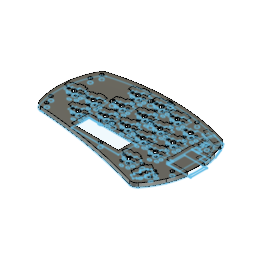
wubmeat-front (Autodesk Fusion 360 design; units mm, degrees)
Autodesk Fusion 360 part; units mm, degrees
(part 1 of 3)
sketch "Sketch1" plane through (0, 0, 0) normal (0, 0, 1) x (1, 0, 0)
  spline S0 degree 3 poles (91.4694, -71.3335) (91.4694, -70.9993) (91.6021, -70.6788) (91.8384, -70.4425) knots 0 0 0 0 1 1 1 1
  line L0 (93.9894, -71.3335) -> (93.9894, -71.3335)
  spline S1 degree 3 poles (103.5273, -74.6924) (103.1931, -74.6924) (102.8726, -74.5596) (102.6363, -74.3233) knots 0 0 0 0 1 1 1 1
  spline S2 degree 3 poles (16.5442, -44.4964) (16.5875, -44.9911) (17.0233, -45.3572) (17.5181, -45.3146) knots 0 0 0 0 1 1 1 1
  line L1 (38.2362, -60.5669) -> (36.9312, -60.6811)
  spline S3 degree 3 poles (61.5612, -48.3605) (61.9831, -48.7824) (62.2202, -49.3547) (62.2202, -49.9515) knots 0 0 0 0 1 1 1 1
  spline S4 degree 3 poles (59.9702, -47.7015) (60.5669, -47.7015) (61.1392, -47.9385) (61.5612, -48.3605) knots 0 0 0 0 1 1 1 1
  spline S5 degree 3 poles (39.0532, -59.592) (39.0099, -59.0973) (38.5741, -58.7311) (38.0794, -58.7738) knots 0 0 0 0 1 1 1 1
  line L2 (38.0794, -58.7738) -> (36.7744, -58.8879)
  spline S6 degree 3 poles (112.7726, -52.689) (113.0089, -52.9253) (113.1417, -53.2458) (113.1417, -53.58) knots 0 0 0 0 1 1 1 1
  spline S7 degree 3 poles (101.7793, -52.3051) (102.0156, -52.5414) (102.1483, -52.8619) (102.1483, -53.1961) knots 0 0 0 0 1 1 1 1
  spline S8 degree 3 poles (59.9702, -52.2015) (59.3735, -52.2015) (58.8012, -51.9644) (58.3792, -51.5425) knots 0 0 0 0 1 1 1 1
  spline S9 degree 3 poles (112.7726, -54.4709) (112.5363, -54.7072) (112.2158, -54.84) (111.8816, -54.84) knots 0 0 0 0 1 1 1 1
  line L3 (113.1417, -53.58) -> (113.1417, -53.58)
  spline S10 degree 3 poles (95.477, -77.878) (95.3823, -78.3656) (95.7004, -78.8377) (96.1878, -78.933) knots 0 0 0 0 1 1 1 1
  spline S11 degree 3 poles (110.6217, -53.58) (110.6217, -53.2458) (110.7544, -52.9253) (110.9907, -52.689) knots 0 0 0 0 1 1 1 1
  spline S12 degree 3 poles (93.6203, -72.2244) (93.384, -72.4607) (93.0635, -72.5935) (92.7294, -72.5935) knots 0 0 0 0 1 1 1 1
  spline S13 degree 3 poles (104.7873, -73.4324) (104.7873, -73.7666) (104.6545, -74.0871) (104.4182, -74.3233) knots 0 0 0 0 1 1 1 1
  spline S14 degree 3 poles (93.6203, -70.4425) (93.8566, -70.6788) (93.9894, -70.9993) (93.9894, -71.3335) knots 0 0 0 0 1 1 1 1
  spline S15 degree 3 poles (102.6363, -74.3233) (102.4, -74.0871) (102.2673, -73.7666) (102.2673, -73.4324) knots 0 0 0 0 1 1 1 1
  spline S16 degree 3 poles (17.3612, -43.5214) (16.8665, -43.5654) (16.5009, -44.0016) (16.5442, -44.4964) knots 0 0 0 0 1 1 1 1
  spline S17 degree 3 poles (111.8816, -54.84) (111.5475, -54.84) (111.227, -54.7072) (110.9907, -54.4709) knots 0 0 0 0 1 1 1 1
  line L4 (18.6662, -43.4073) -> (17.3612, -43.5214)
  spline S18 degree 3 poles (80.6112, -29.3105) (81.0331, -29.7324) (81.2702, -30.3047) (81.2702, -30.9015) knots 0 0 0 0 1 1 1 1
  spline S19 degree 3 poles (110.9907, -52.689) (111.227, -52.4527) (111.5475, -52.32) (111.8816, -52.32) knots 0 0 0 0 1 1 1 1
  spline S20 degree 3 poles (36.7744, -58.8879) (36.2797, -58.9319) (35.9141, -59.3681) (35.9574, -59.8629) knots 0 0 0 0 1 1 1 1
  spline S21 degree 3 poles (104.4182, -74.3233) (104.1819, -74.5596) (103.8614, -74.6924) (103.5273, -74.6924) knots 0 0 0 0 1 1 1 1
  line L5 (18.8231, -45.2004) -> (17.5181, -45.3146)
  spline S22 degree 3 poles (79.0202, -28.6515) (79.6169, -28.6515) (80.1892, -28.8885) (80.6112, -29.3105) knots 0 0 0 0 1 1 1 1
  spline S23 degree 3 poles (92.7294, -70.0735) (93.0635, -70.0735) (93.384, -70.2062) (93.6203, -70.4425) knots 0 0 0 0 1 1 1 1
  spline S24 degree 3 poles (19.6401, -44.2255) (19.5968, -43.7308) (19.161, -43.3646) (18.6662, -43.4073) knots 0 0 0 0 1 1 1 1
  spline S25 degree 3 poles (28.0789, -49.5101) (28.2116, -49.4999) (28.3345, -49.4367) (28.42, -49.3348) knots 0 0 0 0 1 1 1 1
  spline S26 degree 3 poles (38.2362, -60.5669) (38.7309, -60.523) (39.0965, -60.0867) (39.0532, -59.592) knots 0 0 0 0 1 1 1 1
  spline S27 degree 3 poles (81.2702, -30.9015) (81.2702, -31.4982) (81.0331, -32.0705) (80.6112, -32.4925) knots 0 0 0 0 1 1 1 1
  spline S28 degree 3 poles (110.9907, -54.4709) (110.7544, -54.2346) (110.6217, -53.9142) (110.6217, -53.58) knots 0 0 0 0 1 1 1 1
  spline S29 degree 3 poles (61.5612, -51.5425) (61.1392, -51.9644) (60.5669, -52.2015) (59.9702, -52.2015) knots 0 0 0 0 1 1 1 1
  line L6 (62.2202, -49.9515) -> (62.2202, -49.9515)
  spline S30 degree 3 poles (62.2202, -49.9515) (62.2202, -50.5482) (61.9831, -51.1205) (61.5612, -51.5425) knots 0 0 0 0 1 1 1 1
  spline S31 degree 3 poles (80.6112, -32.4925) (80.1892, -32.9144) (79.6169, -33.1515) (79.0202, -33.1515) knots 0 0 0 0 1 1 1 1
  spline S32 degree 3 poles (31.9578, -53.6879) (31.2089, -53.7176) (30.6072, -54.3153) (30.5725, -55.0639) knots 0 0 0 0 1 1 1 1
  spline S33 degree 3 poles (76.7702, -30.9015) (76.7702, -30.3047) (77.0073, -29.7324) (77.4292, -29.3105) knots 0 0 0 0 1 1 1 1
  spline S34 degree 3 poles (111.8816, -52.32) (112.2158, -52.32) (112.5363, -52.4527) (112.7726, -52.689) knots 0 0 0 0 1 1 1 1
  line L7 (102.1483, -53.1961) -> (102.1483, -53.1961)
  spline S35 degree 3 poles (35.9574, -59.8629) (36.0006, -60.3576) (36.4365, -60.7237) (36.9312, -60.6811) knots 0 0 0 0 1 1 1 1
  spline S36 degree 3 poles (102.2673, -73.4324) (102.2673, -73.0982) (102.4, -72.7777) (102.6363, -72.5414) knots 0 0 0 0 1 1 1 1
  spline S37 degree 3 poles (28.42, -49.3348) (28.5055, -49.2329) (28.5464, -49.1008) (28.5335, -48.9684) knots 0 0 0 0 1 1 1 1
  line L8 (33.5517, -53.5485) -> (31.9578, -53.6879)
  spline S38 degree 3 poles (58.3792, -51.5425) (57.9573, -51.1205) (57.7202, -50.5482) (57.7202, -49.9515) knots 0 0 0 0 1 1 1 1
  spline S39 degree 3 poles (58.3792, -48.3605) (58.8012, -47.9385) (59.3735, -47.7015) (59.9702, -47.7015) knots 0 0 0 0 1 1 1 1
  spline S40 degree 3 poles (96.5313, -77.1661) (96.0436, -77.0718) (95.5718, -77.3905) (95.477, -77.878) knots 0 0 0 0 1 1 1 1
  line L9 (97.4738, -79.183) -> (96.1878, -78.933)
  spline S41 degree 3 poles (77.4292, -32.4925) (77.0073, -32.0705) (76.7702, -31.4982) (76.7702, -30.9015) knots 0 0 0 0 1 1 1 1
  spline S42 degree 3 poles (91.8384, -72.2244) (91.6021, -71.9882) (91.4694, -71.6677) (91.4694, -71.3335) knots 0 0 0 0 1 1 1 1
  spline S43 degree 3 poles (91.8384, -70.4425) (92.0747, -70.2062) (92.3952, -70.0735) (92.7294, -70.0735) knots 0 0 0 0 1 1 1 1
  spline S44 degree 3 poles (99.6283, -53.1961) (99.6283, -52.5002) (100.1925, -51.9361) (100.8883, -51.9361) knots 0 0 0 0 1 1 1 1
  spline S45 degree 3 poles (57.7202, -49.9515) (57.7202, -49.3547) (57.9573, -48.7824) (58.3792, -48.3605) knots 0 0 0 0 1 1 1 1
  spline S46 degree 3 poles (79.0202, -33.1515) (78.4235, -33.1515) (77.8512, -32.9144) (77.4292, -32.4925) knots 0 0 0 0 1 1 1 1
  spline S47 degree 3 poles (92.7294, -72.5935) (92.3952, -72.5935) (92.0747, -72.4607) (91.8384, -72.2244) knots 0 0 0 0 1 1 1 1
  spline S48 degree 3 poles (93.9894, -71.3335) (93.9894, -71.6677) (93.8566, -71.9882) (93.6203, -72.2244) knots 0 0 0 0 1 1 1 1
  line L10 (21.1311, -51.2724) -> (23.6963, -51.0479)
  spline S49 degree 3 poles (113.1417, -53.58) (113.1417, -53.9142) (113.0089, -54.2346) (112.7726, -54.4709) knots 0 0 0 0 1 1 1 1
  spline S50 degree 3 poles (77.4292, -29.3105) (77.8512, -28.8885) (78.4235, -28.6515) (79.0202, -28.6515) knots 0 0 0 0 1 1 1 1
  line L11 (81.2702, -30.9015) -> (81.2702, -30.9015)
  line L12 (97.8172, -77.4161) -> (96.5313, -77.1661)
  line L13 (30.6553, -56.0103) -> (30.5725, -55.0639)
  line L14 (78.4006, -7.8462) -> (80.9752, -7.8911)
  line L15 (32.9635, -30.5322) -> (33.0053, -31.0104)
  spline S51 degree 3 poles (88.9155, -11.3802) (88.1676, -11.3315) (87.5067, -11.8629) (87.3939, -12.6039) knots 0 0 0 0 1 1 1 1
  spline S52 degree 3 poles (93.1621, -17.0552) (92.6655, -17.047) (92.2561, -17.4428) (92.2474, -17.9394) knots 0 0 0 0 1 1 1 1
  line L16 (23.6963, -51.0479) -> (23.5961, -49.9023)
  line L17 (94.5104, -10.5778) -> (94.5906, -5.9785)
  line L18 (80.9953, -6.7413) -> (85.4946, -6.8198)
  line L19 (35.9565, -35.3697) -> (35.5556, -30.7872)
  line L20 (22.6156, -38.6951) -> (20.0504, -38.9196)
  line L21 (22.2146, -34.1126) -> (22.1144, -32.967)
  line L22 (19.6494, -34.3371) -> (22.2146, -34.1126)
  spline S53 degree 3 poles (92.2474, -17.9394) (92.2387, -18.436) (92.6341, -18.8458) (93.1307, -18.8549) knots 0 0 0 0 1 1 1 1
  line L23 (22.6984, -39.6415) -> (22.6156, -38.6951)
  line L24 (94.4405, -18.8778) -> (93.1307, -18.8549)
  line L25 (80.8783, -13.4403) -> (80.8949, -12.4904)
  line L26 (33.0053, -31.0104) -> (35.5556, -30.7872)
  line L27 (86.0207, -5.3288) -> (86.5293, -4.8376)
  spline S54 degree 3 poles (94.4405, -18.8778) (94.9371, -18.886) (95.3465, -18.4903) (95.3552, -17.9936) knots 0 0 0 0 1 1 1 1
  line L28 (29.1736, -39.075) -> (22.6984, -39.6415)
  line L29 (91.5286, -4.9249) -> (92.0394, -5.4539)
  line L30 (92.0394, -5.4539) -> (92.031, -5.9338)
  line L31 (86.0032, -6.3286) -> (86.0207, -5.3288)
  line L32 (80.9752, -7.8911) -> (80.9953, -6.7413)
  line L33 (20.0504, -38.9196) -> (19.6494, -34.3371)
  line L34 (24.18, -56.5768) -> (24.0972, -55.6304)
  line L35 (28.4463, -47.9722) -> (28.9008, -47.4306)
  line L36 (91.4808, -10.5249) -> (90.5153, -11.4082)
  line L37 (27.4192, -30.4953) -> (32.4001, -30.0595)
  line L38 (27.0518, -32.0331) -> (26.9646, -31.0369)
  line L39 (34.4451, -47.4675) -> (34.487, -47.9457)
  line L40 (24.0972, -55.6304) -> (21.532, -55.8549)
  spline S55 degree 3 poles (95.3552, -17.9936) (95.3639, -17.497) (94.9685, -17.0872) (94.4719, -17.0781) knots 0 0 0 0 1 1 1 1
  line L41 (33.8818, -46.9948) -> (34.4451, -47.4675)
  line L42 (30.6553, -56.0103) -> (24.18, -56.5768)
  line L43 (21.532, -55.8549) -> (21.1311, -51.2724)
  line L44 (34.4197, -52.5691) -> (33.5517, -53.5485)
  line L45 (78.3203, -12.4455) -> (78.4006, -7.8462)
  line L46 (32.938, -35.6338) -> (32.0701, -36.6132)
  line L47 (29.1736, -39.075) -> (29.0908, -38.1286)
  line L48 (28.9008, -47.4306) -> (33.8818, -46.9948)
  line L49 (28.5335, -48.9684) -> (28.4463, -47.9722)
  line L50 (22.1144, -32.967) -> (26.5973, -32.5748)
  line L51 (35.9565, -35.3697) -> (32.938, -35.6338)
  spline S56 degree 3 poles (35.2927, -41.9526) (34.798, -41.9965) (34.4324, -42.4328) (34.4757, -42.9275) knots 0 0 0 0 1 1 1 1
  line L52 (32.4001, -30.0595) -> (32.9635, -30.5322)
  spline S57 degree 3 poles (30.4762, -36.7526) (29.7273, -36.7823) (29.1256, -37.3799) (29.0908, -38.1286) knots 0 0 0 0 1 1 1 1
  spline S58 degree 3 poles (26.5973, -32.5748) (26.7299, -32.5646) (26.8529, -32.5014) (26.9384, -32.3995) knots 0 0 0 0 1 1 1 1
  line L53 (32.0701, -36.6132) -> (30.4762, -36.7526)
  line L54 (37.4381, -52.305) -> (34.4197, -52.5691)
  spline S59 degree 3 poles (85.4946, -6.8198) (85.6276, -6.8235) (85.7564, -6.7735) (85.8521, -6.6811) knots 0 0 0 0 1 1 1 1
  line L55 (86.5293, -4.8376) -> (91.5286, -4.9249)
  line L56 (23.5961, -49.9023) -> (28.0789, -49.5101)
  line L57 (87.3773, -13.5537) -> (80.8783, -13.4403)
  line L58 (92.031, -5.9338) -> (94.5906, -5.9785)
  spline S60 degree 3 poles (26.9384, -32.3995) (27.0239, -32.2976) (27.0648, -32.1655) (27.0518, -32.0331) knots 0 0 0 0 1 1 1 1
  line L59 (34.487, -47.9457) -> (37.0372, -47.7225)
  line L60 (80.8949, -12.4904) -> (78.3203, -12.4455)
  spline S61 degree 3 poles (85.8521, -6.6811) (85.9478, -6.5887) (86.0023, -6.4617) (86.0032, -6.3286) knots 0 0 0 0 1 1 1 1
  line L61 (94.4719, -17.0781) -> (93.1621, -17.0552)
  line L62 (87.3773, -13.5537) -> (87.3939, -12.6039)
  line L63 (90.5153, -11.4082) -> (88.9155, -11.3802)
  line L64 (94.5104, -10.5778) -> (91.4808, -10.5249)
  line L65 (37.4381, -52.305) -> (37.0372, -47.7225)
  spline S62 degree 3 poles (104.0916, -28.9482) (104.1889, -28.8574) (104.2456, -28.7314) (104.2488, -28.5984) knots 0 0 0 0 1 1 1 1
  line L66 (112.6805, -32.9953) -> (112.8411, -28.3981)
  line L67 (104.8009, -27.1167) -> (109.7978, -27.2912)
  spline S63 degree 3 poles (107.0725, -33.7) (106.3256, -33.6382) (105.6555, -34.1581) (105.5298, -34.8969) knots 0 0 0 0 1 1 1 1
  spline S64 degree 3 poles (37.5716, -42.6567) (37.5283, -42.162) (37.0925, -41.7958) (36.5977, -41.8385) knots 0 0 0 0 1 1 1 1
  line L68 (112.6805, -32.9953) -> (109.6524, -32.8896)
  line L69 (99.0338, -34.6701) -> (96.4603, -34.5802)
  line L70 (96.4603, -34.5802) -> (96.6209, -29.983)
  line L71 (36.5977, -41.8385) -> (35.2927, -41.9526)
  spline S65 degree 3 poles (103.7317, -29.0806) (103.8646, -29.0866) (103.9943, -29.0389) (104.0916, -28.9482) knots 0 0 0 0 1 1 1 1
  line L72 (105.4967, -35.8463) -> (105.5298, -34.8969)
  spline S66 degree 3 poles (34.4757, -42.9275) (34.519, -43.4223) (34.9548, -43.7884) (35.4496, -43.7458) knots 0 0 0 0 1 1 1 1
  line L73 (108.6715, -33.7559) -> (107.0725, -33.7)
  line L74 (110.2994, -27.8291) -> (110.2826, -28.3088)
  line L75 (99.2344, -28.9236) -> (103.7317, -29.0806)
  line L76 (112.5286, -39.494) -> (111.2194, -39.4483)
  spline S67 degree 3 poles (112.4658, -41.2929) (112.9623, -41.3099) (113.3787, -40.9213) (113.396, -40.4248) knots 0 0 0 0 1 1 1 1
  line L77 (112.4658, -41.2929) -> (111.1566, -41.2472)
  spline S68 degree 3 poles (110.2894, -40.3163) (110.2721, -40.8128) (110.6602, -41.2294) (111.1566, -41.2472) knots 0 0 0 0 1 1 1 1
  spline S69 degree 3 poles (113.0591, -24.3032) (113.5556, -24.3202) (113.972, -23.9317) (113.9893, -23.4352) knots 0 0 0 0 1 1 1 1
  spline S70 degree 3 poles (113.9893, -23.4352) (114.0067, -22.9387) (113.6184, -22.522) (113.1219, -22.5043) knots 0 0 0 0 1 1 1 1
  line L78 (110.8759, -11.3191) -> (113.4344, -11.4085)
  line L79 (104.877, -10.6093) -> (105.3942, -10.1271)
  line L80 (109.7978, -27.2912) -> (110.2994, -27.8291)
  spline S71 degree 3 poles (36.7546, -43.6316) (37.2493, -43.5877) (37.6149, -43.1514) (37.5716, -42.6567) knots 0 0 0 0 1 1 1 1
  line L81 (109.6524, -32.8896) -> (108.6715, -33.7559)
  spline S72 degree 3 poles (111.2194, -39.4483) (110.723, -39.4314) (110.3068, -39.8199) (110.2894, -40.3163) knots 0 0 0 0 1 1 1 1
  spline S73 degree 3 poles (113.396, -40.4248) (113.4134, -39.9283) (113.0251, -39.5117) (112.5286, -39.494) knots 0 0 0 0 1 1 1 1
  line L82 (36.7546, -43.6316) -> (35.4496, -43.7458)
  line L83 (113.0591, -24.3032) -> (111.7499, -24.2575)
  line L84 (110.3911, -10.3016) -> (110.8927, -10.8394)
  line L85 (99.8277, -11.9339) -> (104.325, -12.091)
  line L86 (106.0899, -18.8567) -> (99.5939, -18.6299)
  spline S74 degree 3 poles (104.325, -12.091) (104.4579, -12.097) (104.5876, -12.0493) (104.6849, -11.9585) knots 0 0 0 0 1 1 1 1
  spline S75 degree 3 poles (110.8825, -23.3267) (110.8652, -23.8232) (111.2534, -24.2398) (111.7499, -24.2575) knots 0 0 0 0 1 1 1 1
  line L87 (113.2738, -16.0057) -> (113.4344, -11.4085)
  line L88 (106.0899, -18.8567) -> (106.1231, -17.9073)
  line L89 (99.0006, -35.6195) -> (99.0338, -34.6701)
  line L90 (99.5939, -18.6299) -> (99.6271, -17.6804)
  line L91 (97.2142, -12.9934) -> (99.7876, -13.0832)
  line L92 (110.2457, -15.8999) -> (109.2648, -16.7662)
  line L93 (26.9646, -31.0369) -> (27.4192, -30.4953)
  line L94 (105.4967, -35.8463) -> (99.0006, -35.6195)
  line L95 (110.2826, -28.3088) -> (112.8411, -28.3981)
  spline S76 degree 3 poles (107.6658, -16.7104) (106.9189, -16.6486) (106.2488, -17.1684) (106.1231, -17.9073) knots 0 0 0 0 1 1 1 1
  line L96 (99.7876, -13.0832) -> (99.8277, -11.9339)
  line L97 (113.1219, -22.5043) -> (111.8127, -22.4586)
  line L98 (104.2488, -28.5984) -> (104.2837, -27.599)
  line L99 (96.6209, -29.983) -> (99.1943, -30.0729)
  spline S77 degree 3 poles (104.6849, -11.9585) (104.7822, -11.8678) (104.8389, -11.7417) (104.8421, -11.6087) knots 0 0 0 0 1 1 1 1
  line L100 (109.2648, -16.7662) -> (107.6658, -16.7104)
  line L101 (104.2837, -27.599) -> (104.8009, -27.1167)
  line L102 (113.2738, -16.0057) -> (110.2457, -15.8999)
  line L103 (110.8927, -10.8394) -> (110.8759, -11.3191)
  line L104 (97.0536, -17.5906) -> (97.2142, -12.9934)
  spline S78 degree 3 poles (111.8127, -22.4586) (111.3162, -22.4416) (110.8998, -22.8302) (110.8825, -23.3267) knots 0 0 0 0 1 1 1 1
  line L105 (99.6271, -17.6804) -> (97.0536, -17.5906)
  line L106 (99.1943, -30.0729) -> (99.2344, -28.9236)
  spline S79 degree 3 poles (112.1172, -74.4556) (112.0677, -74.3829) (111.9997, -74.3248) (111.9203, -74.2871) knots 0 0 0 0 1 1 1 1
  line L107 (122.6316, -28.9815) -> (118.7816, -28.9815)
  line L108 (118.7816, -28.9815) -> (118.7816, -25.5915)
  spline S80 degree 3 poles (93.8471, -52.8726) (94.3438, -52.8808) (94.7531, -52.4851) (94.7618, -51.9885) knots 0 0 0 0 1 1 1 1
  line L109 (93.8785, -51.0729) -> (92.5687, -51.05)
  line L110 (93.917, -44.5726) -> (90.8874, -44.5197)
  spline S81 degree 3 poles (84.9012, -40.8147) (85.0342, -40.8184) (85.163, -40.7684) (85.2587, -40.6759) knots 0 0 0 0 1 1 1 1
  line L111 (116.1996, -81.9373) -> (115.3459, -81.5208)
  spline S82 degree 3 poles (112.2014, -74.701) (112.1957, -74.6132) (112.1666, -74.5284) (112.1172, -74.4556) knots 0 0 0 0 1 1 1 1
  line L112 (119.0491, -76.0948) -> (116.1996, -81.9373)
  line L113 (111.2113, -79.5044) -> (110.1778, -79)
  line L114 (118.0383, -71.0961) -> (118.4305, -72.3441)
  spline S83 degree 3 poles (117.5933, -74.8209) (117.6795, -75.1722) (117.8944, -75.4783) (118.1954, -75.6788) knots 0 0 0 0 1 1 1 1
  line L115 (112.9833, -68.6859) -> (113.6783, -68.4466)
  line L116 (105.3942, -10.1271) -> (110.3911, -10.3016)
  line L117 (118.4305, -72.3441) -> (117.7292, -73.7822)
  spline S84 degree 3 poles (91.654, -51.9342) (91.6454, -52.4309) (92.0407, -52.8406) (92.5373, -52.8498) knots 0 0 0 0 1 1 1 1
  line L118 (89.9219, -45.403) -> (88.3221, -45.3751)
  spline S85 degree 3 poles (127.7514, -8.5717) (124.8031, -7.6317) (121.8191, -6.8079) (118.8062, -6.1021) knots 0 0 0 0 1 1 1 1
  spline S86 degree 3 poles (127.9715, -8.6379) (127.8982, -8.6158) (127.8248, -8.5937) (127.7514, -8.5717) knots 0 0 0 0 1 1 1 1
  spline S87 degree 3 poles (112.1503, -74.9553) (112.1896, -74.8766) (112.2073, -74.7888) (112.2014, -74.701) knots 0 0 0 0 1 1 1 1
  line L119 (114.2168, -83.8348) -> (110.0827, -81.8184)
  line L120 (85.9359, -38.8324) -> (90.9352, -38.9197)
  spline S88 degree 3 poles (92.5687, -51.05) (92.0721, -51.0419) (91.6627, -51.4376) (91.654, -51.9342) knots 0 0 0 0 1 1 1 1
  line L121 (119.3664, -68.3727) -> (118.0383, -71.0961)
  line L122 (115.2322, -66.3558) -> (115.2322, -66.3558)
  line L123 (122.6316, -28.9815) -> (118.7816, -28.9815)
  line L124 (118.7816, -25.5915) -> (122.6316, -25.5915)
  line L125 (111.0216, -73.8484) -> (110.7912, -73.1802)
  line L126 (90.8874, -44.5197) -> (89.9219, -45.403)
  line L127 (110.7912, -73.1802) -> (112.9833, -68.6859)
  spline S89 degree 3 poles (85.2587, -40.6759) (85.3544, -40.5835) (85.4089, -40.4565) (85.4098, -40.3235) knots 0 0 0 0 1 1 1 1
  line L128 (118.8062, -6.1021) -> (118.8062, -6.1021)
  line L129 (85.4098, -40.3235) -> (85.4273, -39.3236)
  spline S90 degree 3 poles (117.7292, -73.7822) (117.5555, -74.0992) (117.507, -74.4699) (117.5933, -74.8209) knots 0 0 0 0 1 1 1 1
  line L130 (119.8516, -54.0815) -> (119.8516, -37.7315)
  line L131 (118.4516, -54.0665) -> (118.4516, -29.0465)
  line L132 (120.2166, -19.5965) -> (120.2166, -16.4365)
  line L133 (122.6316, -25.5915) -> (122.6316, -28.9815)
  line L134 (115.2322, -66.3558) -> (119.3664, -68.3727)
  line L135 (133.7216, -15.5315) -> (128.9416, -17.3815)
  line L136 (110.1778, -79) -> (112.1503, -74.9553)
  line L137 (114.1098, -68.657) -> (115.2322, -66.3558)
  line L138 (136.3216, -29.0465) -> (136.3216, -33.6665)
  spline S91 degree 3 poles (88.3221, -45.3751) (87.5742, -45.3263) (86.9134, -45.8578) (86.8005, -46.5987) knots 0 0 0 0 1 1 1 1
  line L139 (113.6783, -68.4466) -> (114.1098, -68.657)
  spline S92 degree 3 poles (94.7618, -51.9885) (94.7705, -51.4918) (94.3752, -51.0821) (93.8785, -51.0729) knots 0 0 0 0 1 1 1 1
  line L140 (118.1954, -75.6788) -> (119.0491, -76.0948)
  line L141 (91.4377, -39.9286) -> (93.9973, -39.9733)
  line L142 (104.8421, -11.6087) -> (104.877, -10.6093)
  line L143 (90.9352, -38.9197) -> (91.446, -39.4487)
  line L144 (86.784, -47.5486) -> (80.2849, -47.4351)
  line L145 (86.784, -47.5486) -> (86.8005, -46.5987)
  line L146 (110.0827, -81.8184) -> (111.2113, -79.5044)
  line L147 (93.8471, -52.8726) -> (92.5373, -52.8498)
  line L148 (115.3459, -81.5208) -> (114.2168, -83.8348)
  line L149 (111.9203, -74.2871) -> (111.0216, -73.8484)
  line L150 (118.7816, -28.9815) -> (118.7816, -25.5915)
  line L151 (118.7816, -25.5915) -> (122.6316, -25.5915)
  line L152 (137.2216, -24.2815) -> (133.7216, -15.5315)
  line L153 (119.0516, -48.9015) -> (119.0516, -52.5115)
  line L154 (115.5823, -12.1346) -> (111.6395, -11.0314)
  line L155 (119.8516, -54.0815) -> (119.8516, -37.7315)
  line L156 (123.5816, -25.9315) -> (123.5816, -29.0215)
  line L157 (123.5816, -29.0215) -> (125.0516, -29.0215)
  line L158 (118.6066, -16.4365) -> (118.6066, -19.5965)
  line L159 (116.5981, -7.8464) -> (115.5823, -12.1346)
  line L160 (112.695, -6.8695) -> (116.5981, -7.8464)
  line L161 (131.0416, -33.6665) -> (131.0416, -29.0465)
  line L162 (120.2166, -16.4365) -> (118.6066, -16.4365)
  line L163 (121.8916, -24.6315) -> (121.8916, -21.4715)
  line L164 (121.8916, -24.6315) -> (121.8916, -21.4715)
  line L165 (122.9416, -19.6115) -> (122.9416, -16.4515)
  spline S93 degree 3 poles (50.2132, -44.4132) (49.4637, -44.4168) (48.8415, -44.993) (48.7806, -45.74) knots 0 0 0 0 1 1 1 1
  line L166 (115.0116, -13.2315) -> (117.0316, -5.3565)
  line L167 (121.8916, -21.4715) -> (119.4916, -21.4715)
  line L168 (122.9416, -16.4515) -> (121.3316, -16.4515)
  line L169 (119.4916, -24.6315) -> (121.8916, -24.6315)
  line L170 (119.8516, -37.7315) -> (142.1616, -37.7315)
  line L171 (136.3216, -29.0465) -> (136.3216, -33.6665)
  line L172 (119.0516, -52.5115) -> (116.9616, -52.5115)
  line L173 (136.3216, -33.6665) -> (131.0416, -33.6665)
  line L174 (116.9616, -52.5115) -> (116.9616, -48.9015)
  line L175 (118.6066, -19.5965) -> (120.2166, -19.5965)
  line L176 (116.9616, -48.9015) -> (119.0516, -48.9015)
  line L177 (128.9416, -17.3815) -> (132.3216, -26.0915)
  line L178 (111.6395, -11.0314) -> (112.695, -6.8695)
  line L179 (118.4516, -29.0465) -> (131.1316, -29.0465)
  line L180 (116.9616, -48.9015) -> (119.0516, -48.9015)
  line L181 (119.0516, -52.5115) -> (116.9616, -52.5115)
  line L182 (129.5116, -8.7615) -> (127.3916, -16.5315)
  line L183 (121.3316, -19.6115) -> (122.9416, -19.6115)
  line L184 (127.3916, -16.5315) -> (115.0116, -13.2315)
  line L185 (142.1616, -37.7315) -> (142.1616, -54.0815)
  line L186 (136.3216, -33.6665) -> (131.0416, -33.6665)
  line L187 (131.1316, -54.0665) -> (118.4516, -54.0665)
  line L188 (119.8516, -37.7315) -> (142.1616, -37.7315)
  line L189 (118.6066, -19.5965) -> (120.2166, -19.5965)
  line L190 (131.0416, -29.0465) -> (136.3216, -29.0465)
  line L191 (120.2166, -19.5965) -> (120.2166, -16.4365)
  line L192 (142.1616, -54.0815) -> (119.8516, -54.0815)
  line L193 (131.1316, -54.0665) -> (118.4516, -54.0665)
  line L194 (118.4516, -54.0665) -> (118.4516, -29.0465)
  line L195 (118.4516, -29.0465) -> (131.1316, -29.0465)
  line L196 (119.0516, -48.9015) -> (119.0516, -52.5115)
  line L197 (120.2166, -16.4365) -> (118.6066, -16.4365)
  line L198 (131.0416, -29.0465) -> (136.3216, -29.0465)
  line L199 (117.0316, -5.3565) -> (129.5116, -8.7615)
  line L200 (142.1616, -54.0815) -> (119.8516, -54.0815)
  line L201 (131.1316, -29.0465) -> (131.1316, -54.0665)
  line L202 (125.0516, -29.0215) -> (125.0516, -25.9315)
  line L203 (119.4916, -21.4715) -> (119.4916, -24.6315)
  line L204 (121.3316, -16.4515) -> (121.3316, -19.6115)
  line L205 (125.0516, -25.9315) -> (123.5816, -25.9315)
  line L206 (125.0516, -29.0215) -> (125.0516, -25.9315)
  line L207 (122.9416, -19.6115) -> (122.9416, -16.4515)
  line L208 (48.8304, -46.6887) -> (48.7806, -45.74)
  line L209 (52.9161, -38.2834) -> (52.9412, -38.7627)
  line L210 (132.3216, -26.0915) -> (137.2216, -24.2815)
  line L211 (122.9416, -16.4515) -> (121.3316, -16.4515)
  spline S94 degree 3 poles (46.8294, -39.9393) (46.9185, -39.8404) (46.9639, -39.7099) (46.9556, -39.5771) knots 0 0 0 0 1 1 1 1
  line L212 (42.0488, -41.4865) -> (41.9886, -40.3381)
  line L213 (46.9033, -38.5785) -> (47.3764, -38.053)
  line L214 (39.7181, -46.215) -> (39.4773, -41.6213)
  line L215 (123.5816, -29.0215) -> (125.0516, -29.0215)
  line L216 (121.8916, -21.4715) -> (119.4916, -21.4715)
  line L217 (46.9556, -39.5771) -> (46.9033, -38.5785)
  line L218 (55.7384, -43.2224) -> (55.4977, -38.6287)
  line L219 (55.7384, -43.2224) -> (52.7126, -43.381)
  line L220 (42.2895, -46.0802) -> (39.7181, -46.215)
  line L221 (39.4773, -41.6213) -> (42.0488, -41.4865)
  line L222 (52.7126, -43.381) -> (51.811, -44.3295)
  line L223 (52.3696, -37.7913) -> (52.9161, -38.2834)
  line L224 (48.8304, -46.6887) -> (42.3393, -47.0289)
  line L225 (51.811, -44.3295) -> (50.2132, -44.4132)
  spline S95 degree 3 poles (57.0984, -50.5613) (57.0724, -50.0653) (56.6495, -49.6842) (56.1535, -49.7096) knots 0 0 0 0 1 1 1 1
  spline S96 degree 3 poles (56.2477, -51.5071) (56.7437, -51.4806) (57.1243, -51.0573) (57.0984, -50.5613) knots 0 0 0 0 1 1 1 1
  line L226 (52.9412, -38.7627) -> (55.4977, -38.6287)
  line L227 (41.9886, -40.3381) -> (46.4825, -40.1026)
  line L228 (56.1535, -49.7096) -> (54.8453, -49.7782)
  line L229 (125.0516, -25.9315) -> (123.5816, -25.9315)
  line L230 (121.3316, -19.6115) -> (122.9416, -19.6115)
  line L231 (42.3393, -47.0289) -> (42.2895, -46.0802)
  line L232 (47.3764, -38.053) -> (52.3696, -37.7913)
  spline S97 degree 3 poles (75.73, -32.7747) (76.0515, -32.7747) (76.3487, -32.6031) (76.5094, -32.3247) knots 0 0 0 0 1 1 1 1
  spline S98 degree 3 poles (46.4825, -40.1026) (46.6154, -40.097) (46.7404, -40.0381) (46.8294, -39.9393) knots 0 0 0 0 1 1 1 1
  line L233 (119.4916, -24.6315) -> (121.8916, -24.6315)
  line L234 (75.73, -32.7747) -> (74.42, -32.7747)
  spline S99 degree 3 poles (53.9947, -50.724) (54.0207, -51.2199) (54.4435, -51.6011) (54.9395, -51.5757) knots 0 0 0 0 1 1 1 1
  spline S100 degree 3 poles (76.5094, -31.4247) (76.3487, -31.1462) (76.0515, -30.9747) (75.73, -30.9747) knots 0 0 0 0 1 1 1 1
  spline S101 degree 3 poles (74.42, -30.9747) (74.0985, -30.9747) (73.8013, -31.1462) (73.6406, -31.4247) knots 0 0 0 0 1 1 1 1
  line L235 (126.8594, -71.9436) -> (126.2851, -73.1211)
  spline S102 degree 3 poles (73.6406, -32.3247) (73.8013, -32.6031) (74.0985, -32.7747) (74.42, -32.7747) knots 0 0 0 0 1 1 1 1
  spline S103 degree 3 poles (76.5094, -32.3247) (76.6702, -32.0462) (76.6702, -31.7031) (76.5094, -31.4247) knots 0 0 0 0 1 1 1 1
  line L236 (75.73, -30.9747) -> (74.42, -30.9747)
  spline S104 degree 3 poles (124.6673, -72.332) (124.4501, -72.7786) (124.6358, -73.3167) (125.0821, -73.5344) knots 0 0 0 0 1 1 1 1
  line L237 (56.2477, -51.5071) -> (54.9395, -51.5757)
  spline S105 degree 3 poles (126.445, -70.7402) (125.9982, -70.5224) (125.4594, -70.7079) (125.2415, -71.1546) knots 0 0 0 0 1 1 1 1
  spline S106 degree 3 poles (54.8453, -49.7782) (54.3494, -49.8047) (53.9687, -50.228) (53.9947, -50.724) knots 0 0 0 0 1 1 1 1
  spline S107 degree 3 poles (73.6406, -31.4247) (73.4798, -31.7031) (73.4798, -32.0462) (73.6406, -32.3247) knots 0 0 0 0 1 1 1 1
  spline S108 degree 3 poles (126.8594, -71.9436) (127.0772, -71.4969) (126.8917, -70.9581) (126.445, -70.7402) knots 0 0 0 0 1 1 1 1
  spline S109 degree 3 poles (91.9507, -34.9368) (91.9421, -35.4334) (92.3374, -35.8432) (92.834, -35.8524) knots 0 0 0 0 1 1 1 1
  spline S110 degree 3 poles (125.0821, -73.5344) (125.5285, -73.7521) (126.0668, -73.5671) (126.2851, -73.1211) knots 0 0 0 0 1 1 1 1
  spline S111 degree 3 poles (95.0585, -34.9911) (95.0672, -34.4944) (94.6719, -34.0846) (94.1752, -34.0755) knots 0 0 0 0 1 1 1 1
  spline S112 degree 3 poles (8.6658, -34.1436) (8.7984, -34.1334) (8.9213, -34.0702) (9.0069, -33.9683) knots 0 0 0 0 1 1 1 1
  spline S113 degree 3 poles (12.5447, -38.3214) (11.7958, -38.3511) (11.1941, -38.9488) (11.1593, -39.6974) knots 0 0 0 0 1 1 1 1
  line L238 (2.1188, -40.4884) -> (1.7179, -35.9059)
  line L239 (94.1752, -34.0755) -> (92.8654, -34.0526)
  line L240 (4.7668, -41.2103) -> (4.684, -40.2639)
  line L241 (4.684, -40.2639) -> (2.1188, -40.4884)
  line L242 (94.1438, -35.8752) -> (92.834, -35.8524)
  line L243 (4.1829, -34.5358) -> (8.6658, -34.1436)
  line L244 (125.2415, -71.1546) -> (124.6673, -72.332)
  line L245 (18.025, -36.9385) -> (15.0065, -37.2026)
  line L246 (15.0738, -32.5792) -> (17.6241, -32.356)
  spline S114 degree 3 poles (94.1438, -35.8752) (94.6405, -35.8834) (95.0498, -35.4877) (95.0585, -34.9911) knots 0 0 0 0 1 1 1 1
  spline S115 degree 3 poles (92.8654, -34.0526) (92.3688, -34.0444) (91.9594, -34.4402) (91.9507, -34.9368) knots 0 0 0 0 1 1 1 1
  line L247 (14.4686, -31.6283) -> (15.032, -32.101)
  line L248 (9.1203, -33.6019) -> (9.0331, -32.6057)
  line L249 (11.2421, -40.6438) -> (11.1593, -39.6974)
  line L250 (11.2421, -40.6438) -> (4.7668, -41.2103)
  line L251 (15.0065, -37.2026) -> (14.1386, -38.182)
  line L252 (9.0331, -32.6057) -> (9.4877, -32.0641)
  line L253 (1.7179, -35.9059) -> (4.2831, -35.6814)
  spline S116 degree 3 poles (18.8231, -45.2004) (19.3178, -45.1565) (19.6834, -44.7202) (19.6401, -44.2255) knots 0 0 0 0 1 1 1 1
  line L254 (14.1386, -38.182) -> (12.5447, -38.3214)
  line L255 (96.0276, -46.9727) -> (98.601, -47.0625)
  line L256 (9.4877, -32.0641) -> (14.4686, -31.6283)
  line L257 (4.2831, -35.6814) -> (4.1829, -34.5358)
  line L258 (98.4405, -51.6597) -> (95.867, -51.5699)
  line L259 (18.025, -36.9385) -> (17.6241, -32.356)
  line L260 (112.0872, -49.985) -> (112.2478, -45.3878)
  spline S117 degree 3 poles (66.575, -3.8747) (66.708, -3.876) (66.836, -3.8238) (66.9301, -3.7297) knots 0 0 0 0 1 1 1 1
  spline S118 degree 3 poles (9.0069, -33.9683) (9.0924, -33.8664) (9.1333, -33.7343) (9.1203, -33.6019) knots 0 0 0 0 1 1 1 1
  line L261 (15.032, -32.101) -> (15.0738, -32.5792)
  line L262 (98.4073, -52.6091) -> (98.4405, -51.6597)
  line L263 (104.9034, -52.836) -> (98.4073, -52.6091)
  line L264 (95.867, -51.5699) -> (96.0276, -46.9727)
  line L265 (104.9034, -52.836) -> (104.9365, -51.8866)
  line L266 (112.0872, -49.985) -> (109.0591, -49.8792)
  line L267 (103.6904, -44.5886) -> (104.2076, -44.1064)
  line L268 (98.6411, -45.9132) -> (103.1384, -46.0703)
  spline S119 degree 3 poles (70.075, -8.3747) (69.3264, -8.3389) (68.6749, -8.8819) (68.575, -9.6247) knots 0 0 0 0 1 1 1 1
  line L269 (75.655, -7.4747) -> (72.625, -7.4747)
  line L270 (103.6556, -45.588) -> (103.6904, -44.5886)
  line L271 (109.0591, -49.8792) -> (108.0783, -50.7455)
  line L272 (59.5, -5.0247) -> (62.075, -5.0247)
  line L273 (73.095, -2.3947) -> (73.095, -2.8747)
  line L274 (73.095, -2.8747) -> (75.655, -2.8747)
  line L275 (68.575, -10.5747) -> (68.575, -9.6247)
  line L276 (104.2076, -44.1064) -> (109.2046, -44.2809)
  line L277 (109.7061, -44.8187) -> (109.6893, -45.2984)
  line L278 (67.075, -2.3747) -> (67.575, -1.8747)
  spline S120 degree 3 poles (126.6656, -23.9955) (126.2015, -23.9955) (125.7564, -23.8111) (125.4282, -23.4829) knots 0 0 0 0 1 1 1 1
  line L279 (128.4156, -22.2455) -> (128.4156, -22.2455)
  spline S121 degree 3 poles (74.42, -13.9747) (73.9229, -13.9747) (73.52, -14.3776) (73.52, -14.8747) knots 0 0 0 0 1 1 1 1
  spline S122 degree 3 poles (72.2291, -4.7389) (71.9009, -5.0671) (71.4558, -5.2515) (70.9916, -5.2515) knots 0 0 0 0 1 1 1 1
  line L280 (86.2116, -70.5365) -> (39.3116, -70.5365)
  line L281 (39.3116, -70.5365) -> (39.3116, -52.9465)
  line L282 (62.075, -5.0247) -> (62.075, -3.8747)
  line L283 (72.625, -7.4747) -> (71.675, -8.3747)
  line L284 (39.3116, -52.9465) -> (86.2116, -52.9465)
  line L285 (59.5, -9.6247) -> (59.5, -5.0247)
  line L286 (86.2116, -70.5365) -> (39.3116, -70.5365)
  line L287 (67.075, -3.3747) -> (67.075, -2.3747)
  spline S123 degree 3 poles (75.73, -15.7747) (76.2271, -15.7747) (76.63, -15.3717) (76.63, -14.8747) knots 0 0 0 0 1 1 1 1
  spline S124 degree 3 poles (76.63, -14.8747) (76.63, -14.3776) (76.2271, -13.9747) (75.73, -13.9747) knots 0 0 0 0 1 1 1 1
  spline S125 degree 3 poles (73.52, -14.8747) (73.52, -15.3717) (73.9229, -15.7747) (74.42, -15.7747) knots 0 0 0 0 1 1 1 1
  line L288 (62.075, -10.5747) -> (62.075, -9.6247)
  spline S126 degree 3 poles (124.9156, -22.2455) (124.9156, -21.7813) (125.1, -21.3362) (125.4282, -21.008) knots 0 0 0 0 1 1 1 1
  spline S127 degree 3 poles (72.7416, -3.5015) (72.7416, -3.9656) (72.5573, -4.4107) (72.2291, -4.7389) knots 0 0 0 0 1 1 1 1
  line L289 (86.2116, -52.9465) -> (86.2116, -70.5365)
  line L290 (68.575, -10.5747) -> (62.075, -10.5747)
  line L291 (75.73, -15.7747) -> (74.42, -15.7747)
  line L292 (72.575, -1.8747) -> (73.095, -2.3947)
  line L293 (75.73, -13.9747) -> (74.42, -13.9747)
  spline S128 degree 3 poles (125.4282, -21.008) (125.7564, -20.6798) (126.2015, -20.4955) (126.6656, -20.4955) knots 0 0 0 0 1 1 1 1
  spline S129 degree 3 poles (126.6656, -20.4955) (127.1298, -20.4955) (127.5749, -20.6798) (127.9031, -21.008) knots 0 0 0 0 1 1 1 1
  line L294 (39.3116, -52.9465) -> (86.2116, -52.9465)
  spline S130 degree 3 poles (70.9916, -5.2515) (70.5275, -5.2515) (70.0824, -5.0671) (69.7542, -4.7389) knots 0 0 0 0 1 1 1 1
  line L295 (75.655, -7.4747) -> (75.655, -2.8747)
  spline S131 degree 3 poles (66.9301, -3.7297) (67.0241, -3.6356) (67.0764, -3.5077) (67.075, -3.3747) knots 0 0 0 0 1 1 1 1
  spline S132 degree 3 poles (69.2416, -3.5015) (69.2416, -3.0373) (69.426, -2.5922) (69.7542, -2.264) knots 0 0 0 0 1 1 1 1
  spline S133 degree 3 poles (69.7542, -2.264) (70.0824, -1.9358) (70.5275, -1.7515) (70.9916, -1.7515) knots 0 0 0 0 1 1 1 1
  spline S134 degree 3 poles (127.9031, -21.008) (128.2313, -21.3362) (128.4156, -21.7813) (128.4156, -22.2455) knots 0 0 0 0 1 1 1 1
  spline S135 degree 3 poles (69.7542, -4.7389) (69.426, -4.4107) (69.2416, -3.9656) (69.2416, -3.5015) knots 0 0 0 0 1 1 1 1
  spline S136 degree 3 poles (70.9916, -1.7515) (71.4558, -1.7515) (71.9009, -1.9358) (72.2291, -2.264) knots 0 0 0 0 1 1 1 1
  line L296 (67.575, -1.8747) -> (72.575, -1.8747)
  spline S137 degree 3 poles (125.4282, -23.4829) (125.1, -23.1547) (124.9156, -22.7096) (124.9156, -22.2455) knots 0 0 0 0 1 1 1 1
  line L297 (62.075, -9.6247) -> (59.5, -9.6247)
  spline S138 degree 3 poles (127.9031, -23.4829) (127.5749, -23.8111) (127.1298, -23.9955) (126.6656, -23.9955) knots 0 0 0 0 1 1 1 1
  spline S139 degree 3 poles (128.4156, -22.2455) (128.4156, -22.7096) (128.2313, -23.1547) (127.9031, -23.4829) knots 0 0 0 0 1 1 1 1
  line L298 (62.075, -3.8747) -> (66.575, -3.8747)
  line L299 (39.3116, -70.5365) -> (39.3116, -52.9465)
  line L300 (71.675, -8.3747) -> (70.075, -8.3747)
  line L301 (46.0659, -22.6004) -> (46.0136, -21.6018)
  spline S140 degree 3 poles (45.9397, -22.9626) (46.0287, -22.8637) (46.0742, -22.7332) (46.0659, -22.6004) knots 0 0 0 0 1 1 1 1
  line L302 (41.4496, -30.0522) -> (41.3998, -29.1035)
  spline S141 degree 3 poles (5.5076, -55.5475) (5.9718, -55.5475) (6.4169, -55.7318) (6.7451, -56.06) knots 0 0 0 0 1 1 1 1
  spline S142 degree 3 poles (6.7451, -56.06) (7.0733, -56.3882) (7.2576, -56.8333) (7.2576, -57.2975) knots 0 0 0 0 1 1 1 1
  spline S143 degree 3 poles (44.703, -6.1492) (44.8359, -6.1436) (44.961, -6.0847) (45.05, -5.9859) knots 0 0 0 0 1 1 1 1
  line L303 (41.3998, -29.1035) -> (38.8284, -29.2383)
  spline S144 degree 3 poles (9.5716, -20.2415) (10.0358, -20.2415) (10.4809, -20.4258) (10.8091, -20.754) knots 0 0 0 0 1 1 1 1
  line L304 (55.2638, -32.7329) -> (53.9556, -32.8015)
  spline S145 degree 3 poles (4.2702, -56.06) (4.5984, -55.7318) (5.0435, -55.5475) (5.5076, -55.5475) knots 0 0 0 0 1 1 1 1
  spline S146 degree 3 poles (55.358, -34.5304) (55.8539, -34.5039) (56.2346, -34.0806) (56.2086, -33.5846) knots 0 0 0 0 1 1 1 1
  line L305 (52.0263, -21.3067) -> (52.0515, -21.786)
  line L306 (11.3216, -21.9915) -> (11.3216, -21.9915)
  line L307 (72.7416, -3.5015) -> (72.7416, -3.5015)
  spline S147 degree 3 poles (69.2942, -74.0289) (68.966, -73.7007) (68.7816, -73.2556) (68.7816, -72.7915) knots 0 0 0 0 1 1 1 1
  spline S148 degree 3 poles (53.9556, -32.8015) (53.4596, -32.828) (53.079, -33.2513) (53.105, -33.7473) knots 0 0 0 0 1 1 1 1
  line L308 (41.1591, -24.5098) -> (41.0989, -23.3614)
  spline S149 degree 3 poles (72.2816, -72.7915) (72.2816, -73.2556) (72.0973, -73.7007) (71.7691, -74.0289) knots 0 0 0 0 1 1 1 1
  line L309 (46.4867, -21.0763) -> (51.4798, -20.8146)
  spline S150 degree 3 poles (45.5927, -23.1259) (45.7257, -23.1203) (45.8507, -23.0614) (45.9397, -22.9626) knots 0 0 0 0 1 1 1 1
  spline S151 degree 3 poles (68.7816, -72.7915) (68.7816, -72.3273) (68.966, -71.8822) (69.2942, -71.554) knots 0 0 0 0 1 1 1 1
  line L310 (51.4798, -20.8146) -> (52.0263, -21.3067)
  spline S152 degree 3 poles (5.5076, -59.0475) (5.0435, -59.0475) (4.5984, -58.8631) (4.2702, -58.5349) knots 0 0 0 0 1 1 1 1
  line L311 (47.9406, -29.712) -> (41.4496, -30.0522)
  line L312 (51.8229, -26.4043) -> (50.9213, -27.3528)
  spline S153 degree 3 poles (3.7576, -57.2975) (3.7576, -56.8333) (3.942, -56.3882) (4.2702, -56.06) knots 0 0 0 0 1 1 1 1
  line L313 (80.4019, -40.7361) -> (84.9012, -40.8147)
  line L314 (47.9406, -29.712) -> (47.8909, -28.7633)
  spline S154 degree 3 poles (8.3342, -23.2289) (8.006, -22.9007) (7.8216, -22.4556) (7.8216, -21.9915) knots 0 0 0 0 1 1 1 1
  spline S155 degree 3 poles (53.105, -33.7473) (53.1309, -34.2432) (53.5538, -34.6244) (54.0498, -34.599) knots 0 0 0 0 1 1 1 1
  spline S156 degree 3 poles (4.2702, -58.5349) (3.942, -58.2067) (3.7576, -57.7616) (3.7576, -57.2975) knots 0 0 0 0 1 1 1 1
  line L315 (50.9213, -27.3528) -> (49.3235, -27.4365)
  spline S157 degree 3 poles (72.2291, -2.264) (72.5573, -2.5922) (72.7416, -3.0373) (72.7416, -3.5015) knots 0 0 0 0 1 1 1 1
  line L316 (93.917, -44.5726) -> (93.9973, -39.9733)
  line L317 (55.358, -34.5304) -> (54.0498, -34.599)
  spline S158 degree 3 poles (49.3235, -27.4365) (48.574, -27.44) (47.9518, -28.0163) (47.8909, -28.7633) knots 0 0 0 0 1 1 1 1
  spline S159 degree 3 poles (9.5716, -23.7415) (9.1075, -23.7415) (8.6624, -23.5571) (8.3342, -23.2289) knots 0 0 0 0 1 1 1 1
  spline S160 degree 3 poles (10.8091, -23.2289) (10.4809, -23.5571) (10.0358, -23.7415) (9.5716, -23.7415) knots 0 0 0 0 1 1 1 1
  spline S161 degree 3 poles (10.8091, -20.754) (11.1373, -21.0822) (11.3216, -21.5273) (11.3216, -21.9915) knots 0 0 0 0 1 1 1 1
  spline S162 degree 3 poles (6.7451, -58.5349) (6.4169, -58.8631) (5.9718, -59.0475) (5.5076, -59.0475) knots 0 0 0 0 1 1 1 1
  spline S163 degree 3 poles (48.4337, -10.4598) (47.6843, -10.4633) (47.0621, -11.0396) (47.0012, -11.7866) knots 0 0 0 0 1 1 1 1
  spline S164 degree 3 poles (11.3216, -21.9915) (11.3216, -22.4556) (11.1373, -22.9007) (10.8091, -23.2289) knots 0 0 0 0 1 1 1 1
  spline S165 degree 3 poles (56.2086, -33.5846) (56.1826, -33.0886) (55.7598, -32.7075) (55.2638, -32.7329) knots 0 0 0 0 1 1 1 1
  line L318 (38.5876, -24.6446) -> (41.1591, -24.5098)
  line L319 (54.8487, -26.2457) -> (51.8229, -26.4043)
  line L320 (46.0136, -21.6018) -> (46.4867, -21.0763)
  spline S166 degree 3 poles (7.8216, -21.9915) (7.8216, -21.5273) (8.006, -21.0822) (8.3342, -20.754) knots 0 0 0 0 1 1 1 1
  spline S167 degree 3 poles (7.2576, -57.2975) (7.2576, -57.7616) (7.0733, -58.2067) (6.7451, -58.5349) knots 0 0 0 0 1 1 1 1
  spline S168 degree 3 poles (70.5316, -74.5415) (70.0675, -74.5415) (69.6224, -74.3571) (69.2942, -74.0289) knots 0 0 0 0 1 1 1 1
  spline S169 degree 3 poles (69.2942, -71.554) (69.6224, -71.2258) (70.0675, -71.0415) (70.5316, -71.0415) knots 0 0 0 0 1 1 1 1
  line L321 (85.4273, -39.3236) -> (85.9359, -38.8324)
  line L322 (77.8072, -41.841) -> (80.3818, -41.886)
  line L323 (7.2576, -57.2975) -> (7.2576, -57.2975)
  line L324 (80.2849, -47.4351) -> (80.3015, -46.4853)
  line L325 (91.446, -39.4487) -> (91.4377, -39.9286)
  line L326 (80.3818, -41.886) -> (80.4019, -40.7361)
  spline S170 degree 3 poles (71.7691, -74.0289) (71.4409, -74.3571) (70.9958, -74.5415) (70.5316, -74.5415) knots 0 0 0 0 1 1 1 1
  line L327 (80.3015, -46.4853) -> (77.7269, -46.4403)
  line L328 (52.0515, -21.786) -> (54.608, -21.652)
  line L329 (38.8284, -29.2383) -> (38.5876, -24.6446)
  spline S171 degree 3 poles (8.3342, -20.754) (8.6624, -20.4258) (9.1075, -20.2415) (9.5716, -20.2415) knots 0 0 0 0 1 1 1 1
  line L330 (77.7269, -46.4403) -> (77.8072, -41.841)
  line L331 (41.0989, -23.3614) -> (45.5927, -23.1259)
  line L332 (54.8487, -26.2457) -> (54.608, -21.652)
  line L333 (67.075, -36.3747) -> (67.575, -35.8747)
  line L334 (40.2092, -6.3847) -> (44.703, -6.1492)
  line L335 (62.075, -43.6247) -> (59.5, -43.6247)
  line L336 (45.597, -4.0996) -> (50.5901, -3.8379)
  line L337 (50.5901, -3.8379) -> (51.1366, -4.33)
  line L338 (37.6979, -7.6679) -> (40.2694, -7.5331)
  line L339 (68.575, -44.5747) -> (68.575, -43.6247)
  spline S172 degree 3 poles (73.6406, -49.3247) (73.8013, -49.6031) (74.0985, -49.7747) (74.42, -49.7747) knots 0 0 0 0 1 1 1 1
  spline S173 degree 3 poles (76.5094, -48.4247) (76.3487, -48.1462) (76.0515, -47.9747) (75.73, -47.9747) knots 0 0 0 0 1 1 1 1
  spline S174 degree 3 poles (45.05, -5.9859) (45.139, -5.887) (45.1845, -5.7565) (45.1762, -5.6237) knots 0 0 0 0 1 1 1 1
  line L340 (50.0315, -10.3761) -> (48.4337, -10.4598)
  line L341 (37.9387, -12.2616) -> (37.6979, -7.6679)
  line L342 (40.5598, -13.0755) -> (40.5101, -12.1268)
  line L343 (54.4683, -17.5537) -> (53.1601, -17.6223)
  line L344 (53.959, -9.269) -> (50.9331, -9.4276)
  line L345 (54.3741, -15.7562) -> (53.0659, -15.8248)
  line L346 (73.095, -36.3947) -> (73.095, -36.8747)
  spline S175 degree 3 poles (70.075, -42.3747) (69.3264, -42.3389) (68.6749, -42.8819) (68.575, -43.6247) knots 0 0 0 0 1 1 1 1
  line L347 (71.675, -42.3747) -> (70.075, -42.3747)
  line L348 (62.075, -39.0247) -> (62.075, -37.8747)
  line L349 (75.73, -49.7747) -> (74.42, -49.7747)
  line L350 (67.075, -37.3747) -> (67.075, -36.3747)
  line L351 (51.1618, -4.8093) -> (53.7182, -4.6753)
  line L352 (73.095, -36.8747) -> (75.655, -36.8747)
  line L353 (62.075, -44.5747) -> (62.075, -43.6247)
  spline S176 degree 3 poles (75.73, -49.7747) (76.0515, -49.7747) (76.3487, -49.6031) (76.5094, -49.3247) knots 0 0 0 0 1 1 1 1
  line L354 (72.625, -41.4747) -> (71.675, -42.3747)
  line L355 (62.075, -37.8747) -> (66.575, -37.8747)
  spline S177 degree 3 poles (73.6406, -48.4247) (73.4798, -48.7031) (73.4798, -49.0462) (73.6406, -49.3247) knots 0 0 0 0 1 1 1 1
  line L356 (40.2694, -7.5331) -> (40.2092, -6.3847)
  line L357 (50.9331, -9.4276) -> (50.0315, -10.3761)
  line L358 (45.1238, -4.6251) -> (45.597, -4.0996)
  spline S178 degree 3 poles (74.42, -47.9747) (74.0985, -47.9747) (73.8013, -48.1462) (73.6406, -48.4247) knots 0 0 0 0 1 1 1 1
  spline S179 degree 3 poles (96.0664, -64.6474) (96.1968, -64.6741) (96.3323, -64.6473) (96.4426, -64.5729) knots 0 0 0 0 1 1 1 1
  spline S180 degree 3 poles (96.4426, -64.5729) (96.5529, -64.4985) (96.6286, -64.3828) (96.6527, -64.252) knots 0 0 0 0 1 1 1 1
  line L359 (68.575, -44.5747) -> (62.075, -44.5747)
  line L360 (40.5101, -12.1268) -> (37.9387, -12.2616)
  line L361 (75.655, -41.4747) -> (75.655, -36.8747)
  line L362 (90.552, -69.4331) -> (88.0243, -68.9418)
  line L363 (47.0509, -12.7353) -> (40.5598, -13.0755)
  line L364 (47.0509, -12.7353) -> (47.0012, -11.7866)
  spline S181 degree 3 poles (98.6435, -69.7326) (97.9154, -69.5546) (97.1723, -69.9633) (96.9325, -70.6734) knots 0 0 0 0 1 1 1 1
  spline S182 degree 3 poles (52.2152, -16.7706) (52.2412, -17.2665) (52.6641, -17.6477) (53.1601, -17.6223) knots 0 0 0 0 1 1 1 1
  spline S183 degree 3 poles (76.5094, -49.3247) (76.6702, -49.0462) (76.6702, -48.7031) (76.5094, -48.4247) knots 0 0 0 0 1 1 1 1
  line L365 (104.2927, -69.9138) -> (101.3184, -69.3357)
  spline S184 degree 3 poles (101.8401, -76.0587) (101.3523, -75.9642) (100.8802, -76.2828) (100.7854, -76.7705) knots 0 0 0 0 1 1 1 1
  line L366 (102.3378, -63.829) -> (102.749, -64.4387)
  line L367 (104.2927, -69.9138) -> (105.1704, -65.3983)
  line L368 (90.3707, -70.3657) -> (90.552, -69.4331)
  spline S185 degree 3 poles (66.575, -37.8747) (66.708, -37.876) (66.836, -37.8238) (66.9301, -37.7297) knots 0 0 0 0 1 1 1 1
  line L369 (75.73, -47.9747) -> (74.42, -47.9747)
  line L370 (67.575, -35.8747) -> (72.575, -35.8747)
  line L371 (72.575, -35.8747) -> (73.095, -36.3947)
  line L372 (88.902, -64.4263) -> (91.4297, -64.9176)
  line L373 (45.1762, -5.6237) -> (45.1238, -4.6251)
  line L374 (51.1366, -4.33) -> (51.1618, -4.8093)
  spline S186 degree 3 poles (53.0659, -15.8248) (52.5699, -15.8513) (52.1892, -16.2746) (52.2152, -16.7706) knots 0 0 0 0 1 1 1 1
  line L375 (53.959, -9.269) -> (53.7182, -4.6753)
  spline S187 degree 3 poles (54.4683, -17.5537) (54.9642, -17.5272) (55.3449, -17.1039) (55.3189, -16.6079) knots 0 0 0 0 1 1 1 1
  spline S188 degree 3 poles (55.3189, -16.6079) (55.2929, -16.1119) (54.8701, -15.7308) (54.3741, -15.7562) knots 0 0 0 0 1 1 1 1
  line L376 (75.655, -41.4747) -> (72.625, -41.4747)
  spline S189 degree 3 poles (66.9301, -37.7297) (67.0241, -37.6356) (67.0764, -37.5077) (67.075, -37.3747) knots 0 0 0 0 1 1 1 1
  line L377 (59.5, -43.6247) -> (59.5, -39.0247)
  line L378 (59.5, -39.0247) -> (62.075, -39.0247)
  spline S190 degree 3 poles (109.6959, -57.306) (109.6786, -57.8025) (110.0668, -58.2191) (110.5633, -58.2368) knots 0 0 0 0 1 1 1 1
  line L379 (31.9567, -46.1594) -> (30.6516, -46.2736)
  line L380 (109.6893, -45.2984) -> (112.2478, -45.3878)
  spline S191 degree 3 poles (31.9567, -46.1594) (32.4513, -46.1155) (32.817, -45.6792) (32.7737, -45.1845) knots 0 0 0 0 1 1 1 1
  line L381 (102.6575, -64.9098) -> (105.1704, -65.3983)
  spline S192 degree 3 poles (103.8374, -77.3638) (103.9322, -76.876) (103.6138, -76.4037) (103.1261, -76.3087) knots 0 0 0 0 1 1 1 1
  line L382 (88.0243, -68.9418) -> (88.902, -64.4263)
  line L383 (96.7513, -71.6059) -> (96.9325, -70.6734)
  spline S193 degree 3 poles (32.7737, -45.1845) (32.7304, -44.6897) (32.2946, -44.3236) (31.7998, -44.3662) knots 0 0 0 0 1 1 1 1
  line L384 (91.4297, -64.9176) -> (91.6491, -63.7888)
  line L385 (101.3184, -69.3357) -> (100.2141, -70.0378)
  spline S194 degree 3 poles (103.1384, -46.0703) (103.2713, -46.0763) (103.401, -46.0285) (103.4983, -45.9378) knots 0 0 0 0 1 1 1 1
  spline S195 degree 3 poles (7.9042, -63.864) (8.2324, -63.5358) (8.6775, -63.3515) (9.1416, -63.3515) knots 0 0 0 0 1 1 1 1
  line L386 (10.8916, -65.1015) -> (10.8916, -65.1015)
  line L387 (102.7826, -78.0756) -> (101.4967, -77.8257)
  spline S196 degree 3 poles (9.1416, -63.3515) (9.6058, -63.3515) (10.0509, -63.5358) (10.3791, -63.864) knots 0 0 0 0 1 1 1 1
  line L388 (109.2046, -44.2809) -> (109.7061, -44.8187)
  spline S197 degree 3 poles (29.6777, -45.4553) (29.721, -45.9501) (30.1569, -46.3162) (30.6516, -46.2736) knots 0 0 0 0 1 1 1 1
  spline S198 degree 3 poles (37.4506, -38.963) (37.4506, -39.2972) (37.3178, -39.6177) (37.0815, -39.854) knots 0 0 0 0 1 1 1 1
  spline S199 degree 3 poles (111.8725, -58.2825) (112.369, -58.2995) (112.7854, -57.911) (112.8027, -57.4145) knots 0 0 0 0 1 1 1 1
  spline S200 degree 3 poles (35.2996, -39.854) (35.0633, -39.6177) (34.9306, -39.2972) (34.9306, -38.963) knots 0 0 0 0 1 1 1 1
  spline S201 degree 3 poles (35.2996, -38.072) (35.5359, -37.8358) (35.8564, -37.703) (36.1906, -37.703) knots 0 0 0 0 1 1 1 1
  spline S202 degree 3 poles (34.9306, -38.963) (34.9306, -38.6288) (35.0633, -38.3083) (35.2996, -38.072) knots 0 0 0 0 1 1 1 1
  spline S203 degree 3 poles (26.4924, -39.9217) (26.4924, -40.2559) (26.3597, -40.5764) (26.1234, -40.8127) knots 0 0 0 0 1 1 1 1
  spline S204 degree 3 poles (24.3415, -40.8127) (24.1052, -40.5764) (23.9724, -40.2559) (23.9724, -39.9217) knots 0 0 0 0 1 1 1 1
  line L389 (108.0783, -50.7455) -> (106.4792, -50.6897)
  spline S205 degree 3 poles (100.7854, -76.7705) (100.6906, -77.2583) (101.009, -77.7306) (101.4967, -77.8257) knots 0 0 0 0 1 1 1 1
  spline S206 degree 3 poles (30.4948, -44.4804) (30.0001, -44.5243) (29.6345, -44.9606) (29.6777, -45.4553) knots 0 0 0 0 1 1 1 1
  line L390 (96.7513, -71.6059) -> (90.3707, -70.3657)
  line L391 (98.601, -47.0625) -> (98.6411, -45.9132)
  spline S207 degree 3 poles (102.7826, -78.0756) (103.2704, -78.1702) (103.7426, -77.8516) (103.8374, -77.3638) knots 0 0 0 0 1 1 1 1
  line L392 (37.4506, -38.963) -> (37.4506, -38.963)
  spline S208 degree 3 poles (25.2324, -38.6617) (25.5666, -38.6617) (25.8871, -38.7945) (26.1234, -39.0308) knots 0 0 0 0 1 1 1 1
  spline S209 degree 3 poles (23.9724, -39.9217) (23.9724, -39.5875) (24.1052, -39.2671) (24.3415, -39.0308) knots 0 0 0 0 1 1 1 1
  spline S210 degree 3 poles (24.3415, -39.0308) (24.5778, -38.7945) (24.8982, -38.6617) (25.2324, -38.6617) knots 0 0 0 0 1 1 1 1
  spline S211 degree 3 poles (37.0815, -39.854) (36.8452, -40.0903) (36.5247, -40.223) (36.1906, -40.223) knots 0 0 0 0 1 1 1 1
  spline S212 degree 3 poles (110.6261, -56.4379) (110.1296, -56.4209) (109.7133, -56.8095) (109.6959, -57.306) knots 0 0 0 0 1 1 1 1
  line L393 (111.8725, -58.2825) -> (110.5633, -58.2368)
  spline S213 degree 3 poles (36.1906, -37.703) (36.5247, -37.703) (36.8452, -37.8358) (37.0815, -38.072) knots 0 0 0 0 1 1 1 1
  spline S214 degree 3 poles (32.7715, -39.4424) (32.7715, -39.9887) (32.5545, -40.5127) (32.1681, -40.899) knots 0 0 0 0 1 1 1 1
  spline S215 degree 3 poles (26.1234, -40.8127) (25.8871, -41.049) (25.5666, -41.1817) (25.2324, -41.1817) knots 0 0 0 0 1 1 1 1
  spline S216 degree 3 poles (25.2324, -41.1817) (24.8982, -41.1817) (24.5778, -41.049) (24.3415, -40.8127) knots 0 0 0 0 1 1 1 1